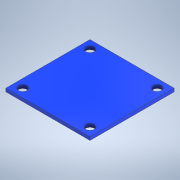
# Autodesk Inventor part: arena_top_bottom
Saved by Autodesk Inventor 2021 (Build 250183000, 183)
## iProperties
Created: 2021-02-15
Part Number: arena_top_bottom
Material: Generic
Document SubType Name: Modeling
Designer: lobato
Density: 1 g/cm^3
Appearance: Default
Author: lobato
Autodesk Inventor part; units mm, degrees
ref_plane "YZ Plane" through (0, 0, 0) normal (1, 0, 0) x (0, 1, 0)
ref_plane "XZ Plane" through (0, 0, 0) normal (0, 1, 0) x (-1, 0, 0)
ref_plane "XY Plane" through (0, 0, 0) normal (0, 0, 1) x (1, 0, 0)
sketch "Sketch1" plane through (0, 0, 0) normal (0, 1, 0) x (-1, 0, 0)
  line L0 (25, 25) -> (-25, 25)
  line L1 (-25, 25) -> (-25, -25)
  line L2 (-25, -25) -> (25, -25)
  line L3 (25, -25) -> (25, 25)
  line L4 (25, 25) -> (-25, -25) construction
  line L5 (-25, 25) -> (25, -25) construction
  line L6 (20, 20) -> (-20, 20) construction
  line L7 (-20, 20) -> (-20, -20) construction
  line L8 (-20, -20) -> (20, -20) construction
  line L9 (20, -20) -> (20, 20) construction
  line L10 (20, 20) -> (-20, -20) construction
  line L11 (-20, 20) -> (20, -20) construction
  circle A0 centre (20, 20) radius 2.55
  circle A1 centre (20, -20) radius 2.55
  circle A2 centre (-20, -20) radius 2.55
  circle A3 centre (-20, 20) radius 2.55
  point P0 (0, 0)
  dimension "d0" = 50
  dimension "d1" = 50
  dimension "d2" = 40
  dimension "d3" = 40
  dimension "d4" = 5.1
  dimension "d5" = 5.1
  dimension "d6" = 5.1
  dimension "d7" = 5.1
  constraints: 24 end point, 4 centre point, 4 coincident, 4 midpoint, 4 parallel, 2 horizontal, 2 perpendicular
  measures "d0" distance of L2.end L1.end
  measures "d1" distance of L1.end L0.end
  measures "d2" distance of L8.end L7.end
  measures "d3" distance of L7.end L6.end
  measures "d4" diameter of A0
  measures "d5" diameter of A1
  measures "d6" diameter of A2
  measures "d7" diameter of A3
extrude "Extrusion1" add sketch "Sketch1" along normal blind 2
body "Solid1"
